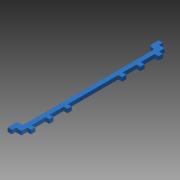
# Autodesk Inventor part: base_support
Saved by Autodesk Inventor 2015 (Build 190159000, 159)
## iProperties
Created: 2015-12-01
Part Number: base_support
Material: Generic
Document SubType Name: Modeling
Designer: jufranz
Density: 1 g/cm^3
Appearance: Cyan
Author: jufranz
Autodesk Inventor part; units mm, degrees
ref_plane "YZ Plane" through (0, 0, 0) normal (1, 0, 0) x (0, 1, 0)
ref_plane "XZ Plane" through (0, 0, 0) normal (0, 1, 0) x (-1, 0, 0)
ref_plane "XY Plane" through (0, 0, 0) normal (0, 0, 1) x (1, 0, 0)
sketch "Sketch1" plane through (0, 0, 0) normal (0, 1, 0) x (-1, 0, 0)
  line L0 (7, 100) -> (-7, 100)
  line L1 (-7, 100) -> (-7, -100)
  line L2 (-7, -100) -> (7, -100)
  line L3 (7, -100) -> (7, 100)
  point P0 (0, 0)
  point P1 (7, 0)
  point P2 (0, 100)
  dimension "d0" = 14
  dimension "d1" = 200
  constraints: 8 end point, 2 midpoint, 2 parallel, 1 horizontal, 1 horizontal alignment, 1 perpendicular, 1 vertical alignment
  measures "d0" distance of L0.start L0.end
  measures "d1" distance of L2.end L0.start
extrude "Extrusion1" add sketch "Sketch1" along normal blind 5.334
sketch "Sketch2" plane through (0, 5.334, 0) normal (0, 1, 0) x (1, 0, 0)
  line L0 (-7, -92) -> (1, -92)
  line L1 (1, -92) -> (1, 92)
  line L2 (1, 92) -> (-7, 92)
  line L3 (-7, 92) -> (-7, -92)
  line L4 (-7, 100) -> (-7, -100) projected
  line L5 (7, -100) -> (7, 100) projected
  line L6 (-7, -100) -> (7, -100) projected
  line L7 (7, 100) -> (-7, 100) projected
  point P0 (0, 0)
  point P1 (-7, 0)
  dimension "d4" = 6
  dimension "d5" = 8
  dimension "d6" = 8
  constraints: 8 end point, 2 midpoint, 2 parallel, 1 horizontal, 1 perpendicular
  measures "d4" distance between parallel lines of L5 L1
  measures "d5" distance between parallel lines of L6 L0
  measures "d6" distance between parallel lines of L7 L2
extrude "Extrusion2" cut sketch "Sketch2" against normal through all contours L3 L2 L1 L0
sketch "Sketch3" plane through (-7, 0, 100) normal (0, 0, 1) x (1, 0, 0)
  line L0 (0, 0) -> (6, 0)
  line L1 (6, 0) -> (6, 5.334)
  line L2 (6, 5.334) -> (0, 5.334)
  line L3 (0, 5.334) -> (0, 0)
  line L4 (0, 5.334) -> (14, 5.334) projected
  point P0 (7, 0)
  point P1 (7, 5.334)
  dimension "d9" = 6
  constraints: 8 end point, 2 parallel, 1 horizontal, 1 midpoint, 1 perpendicular, 1 point on line
  measures "d9" distance between parallel lines of L3 L1
extrude "Extrusion3" add sketch "Sketch3" along normal blind 5.334
sketch "Sketch4" plane through (7, 0, 100) normal (1, 0, 0) x (0, 0, -1)
  line L0 (0, 5.334) -> (200, 5.334) projected
  line L1 (0, 0) -> (200, 0) projected
  line L2 (8, 5.334) -> (14, 5.334)
  line L3 (14, 5.334) -> (14, 0)
  line L4 (14, 0) -> (8, 0)
  line L5 (8, 0) -> (8, 5.334)
  line L6 (0, 0) -> (0, 5.334) projected
  point P0 (100, 0)
  dimension "d13" = 8
  dimension "d14" = 6
  constraints: 8 end point, 2 parallel, 2 point on line, 1 horizontal, 1 perpendicular
  measures "d13" distance between parallel lines of L6 L5
  measures "d14" distance between parallel lines of L5 L3
extrude "Extrusion4" add sketch "Sketch4" along normal blind 5.334 contours L0 L3 L1 L5
pattern_linear "Rectangular Pattern1" count 3 spacing 25.4 along (0, 0, -1) of "Extrusion4"
mirror "Mirror1" about plane through (0, 0, 0) normal (0, 0, 1) of "Extrusion3", "Extrusion4", "Rectangular Pattern1"
fillet "Fillet2" radius 3.175 4 edges at (-7, 2.667, 92) (1, 2.667, 92) (-7, 2.667, -92) (1, 2.667, -92)
equation "\"d6\" = d5"
body "Solid1"
